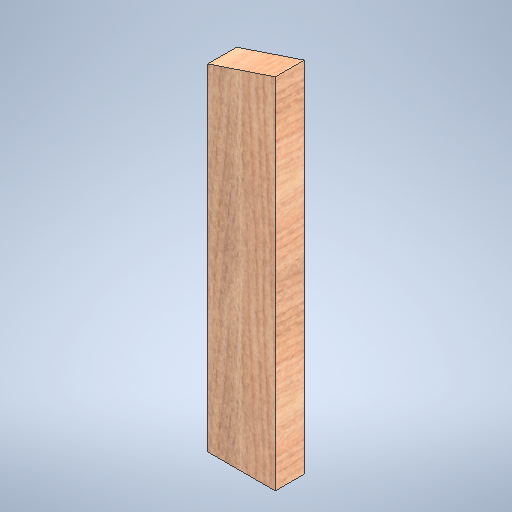
# Autodesk Inventor part: Stud_With_Height_42.5_Inches
Saved by Autodesk Inventor 2025.1 (Build 291241020, 241B)
## iProperties
Created: 2024-09-16
Part Number: Stud_With_Height_42.5_Inches
Material: Wood (Birch)
Document SubType Name: Modeling
Designer: Tom
Density: 0.55 g/cm^3
Appearance: Birch - Natural Polished
Author: Tom
Autodesk Inventor part; units mm, degrees
ref_plane "YZ Plane" through (0, 0, 0) normal (1, 0, 0) x (0, 1, 0)
ref_plane "XZ Plane" through (0, 0, 0) normal (0, 1, 0) x (-1, 0, 0)
ref_plane "XY Plane" through (0, 0, 0) normal (0, 0, 1) x (1, 0, 0)
sketch "Sketch1" plane through (0, 0, 0) normal (0, 0, 1) x (1, 0, 0)
  line L0 (0, 0) -> (88.9, 0)
  line L1 (88.9, 0) -> (88.9, 471.7859)
  line L2 (0, 442.1238) -> (0, 0)
  line L3 (88.9, 471.7859) -> (0, 442.1238)
  line L4 (88.9, 471.7859) -> (-3175, 471.7859)
  line L5 (-3175, 471.7859) -> (-3175, -617.2391)
  line L6 (-3175, -617.2391) -> (88.9, 471.7859)
  dimension "d3" = 88.9
  dimension "d6" = 471.786
  dimension "d9" = 3263.9
  dimension "d10" = 1089.025
  constraints: 14 end point, 2 horizontal, 2 perpendicular, 1 collinear, 1 parallel
  measures "d3" distance of L0.start L0.end
  measures "d6" distance of L0.end L1.end
  measures "d9" distance of L1.end L4.end
  measures "d10" distance of L4.end L5.end
extrude "Extrusion1" add sketch "Sketch1" along normal blind 38.1 contours L2 L3 L1 L0
body "Solid1"
